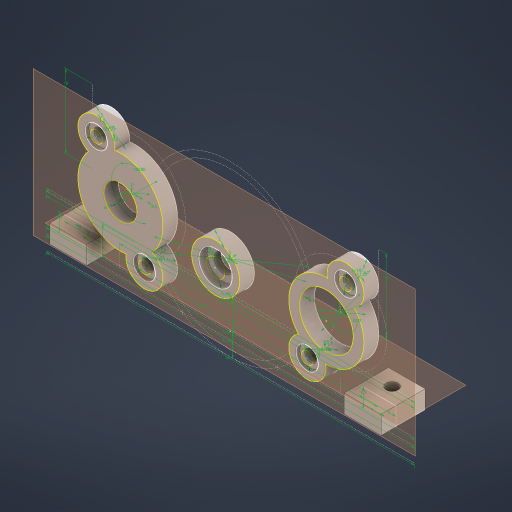
# Autodesk Inventor part: Motormount
Saved by Autodesk Inventor 2023.4 (Build 274418000, 418)
## iProperties
Created: 2024-12-07
Part Number: Motormount
Material: 一般
Document SubType Name: Modeling
Designer: IshiiLabHonda
Density: 1 g/cm^3
Appearance: 既定
Author: IshiiLabHonda
Autodesk Inventor part; units mm, degrees
ref_plane "YZ Plane" through (0, 0, 0) normal (1, 0, 0) x (0, 1, 0)
ref_plane "XZ Plane" through (0, 0, 0) normal (0, 1, 0) x (-1, 0, 0)
ref_plane "XY Plane" through (0, 0, 0) normal (0, 0, 1) x (1, 0, 0)
sketch "blueprint" plane through (0, 0, 0) normal (0, 0, 1) x (1, 0, 0)
  line L0 (0, 0) -> (0, 1) construction
  line L1 (0, 0) -> (1, 0) construction
  circle A0 centre (0, 0) radius 1.25
  circle A1 centre (0, 0) radius 11.5 construction
  line L2 (-25, -11.5) -> (25, -11.5) construction
  line L3 (-25, -9.5) -> (25, -9.5) construction
  line L4 (-25, -8.5) -> (25, -8.5) construction
  line L5 (-25, -4.5) -> (25, -4.5) construction
  circle A2 centre (0, 0) radius 10.65 construction
  circle A3 centre (-12.9388, 1.26) radius 2.25
  circle A4 centre (15.0473, 1.26) radius 4.35 construction
  circle A5 centre (15.0473, 1.26) radius 3.6 construction
  line L6 (-25, -4.1) -> (25, -4.1) construction
  circle A6 centre (-12.9388, 1.26) radius 4.26 construction
  circle A7 centre (-12.9388, 1.26) radius 5.76
  circle A8 centre (-16.1988, 7.3243) radius 0.625 construction
  circle A9 centre (-9.6788, -4.8043) radius 0.625 construction
  circle A10 centre (-12.9388, 1.26) radius 6.885 construction
  circle A11 centre (-16.1988, 7.3243) radius 1.825 construction
  circle A12 centre (-9.6788, -4.8043) radius 1.825 construction
  circle A13 centre (15.0473, 1.26) radius 5.1
  circle A14 centre (15.0473, 1.26) radius 6.225 construction
  circle A15 centre (17.6473, 6.916) radius 0.625 construction
  circle A16 centre (12.4473, -4.396) radius 0.625 construction
  circle A17 centre (17.6473, 6.916) radius 1.825 construction
  circle A18 centre (-16.1988, 7.3243) radius 0.8
  circle A19 centre (-9.6788, -4.8043) radius 0.8
  circle A20 centre (12.4473, -4.396) radius 0.8
  circle A21 centre (17.6473, 6.916) radius 0.8
  circle A22 centre (-16.1988, 7.3243) radius 2.5
  circle A23 centre (-9.6788, -4.8043) radius 2.5
  circle A24 centre (17.6473, 6.916) radius 2.5
  circle A25 centre (12.4473, -4.396) radius 2.5
  circle A26 centre (15.0473, 1.26) radius 3.65
  circle A27 centre (0, 0) radius 3.25
  line L7 (-12.9388, 1.26) -> (-12.9388, 2.26) construction
  line L8 (-12.9388, 1.26) -> (-11.9388, 1.26) construction
  line L9 (15.0473, 1.26) -> (15.0473, 2.26) construction
  line L10 (15.0473, 1.26) -> (16.0473, 1.26) construction
  line L11 (-15, -4.5) -> (-15, -8.5) construction
  line L12 (15, -4.5) -> (15, -8.5) construction
  line L13 (-12.9388, 1.26) -> (15.0473, 1.26) construction
  line L14 (-17.5, -8.5) -> (-17.5, -6)
  line L15 (-22.5, -8.5) -> (-22.5, -6)
  line L16 (-22.5, -6) -> (-17.5, -6)
  line L17 (-20, -6) -> (-20, -8.5)
  line L18 (-21, -6) -> (-21, -8.5)
  line L19 (-19, -6) -> (-19, -8.5)
  line L20 (17.5, -8.5) -> (17.5, -6)
  line L21 (22.5, -8.5) -> (22.5, -6)
  line L22 (22.5, -6) -> (17.5, -6)
  line L23 (20, -6) -> (20, -8.5)
  line L24 (21, -6) -> (21, -8.5)
  line L25 (19, -6) -> (19, -8.5)
  line L26 (-22.5, -8.5) -> (-17.5, -8.5)
  line L27 (17.5, -8.5) -> (22.5, -8.5)
  circle A28 centre (12.4473, -4.396) radius 1.825 construction
  line L28 (-12.9388, 1.26) -> (-16.1988, 7.3243) construction
  line L29 (-12.9388, 1.26) -> (-9.6788, -4.8043) construction
  line L30 (15.0473, 1.26) -> (12.4473, -4.396) construction
  line L31 (-18.6988, 11.26) -> (-18.6988, 1.26) construction
  line L32 (20.1473, 11.26) -> (20.1473, 1.26) construction
  line L33 (17.6473, 6.916) -> (15.0473, 1.26) construction
  point P0 (-8.6127, -2.543)
  point P1 (18.8099, 4.7028)
  point P2 (11.2847, -2.1828)
  point P3 (15.2106, 6.3574)
  point P4 (-12.153, -4.4461)
  point P5 (-13.7246, 6.9661)
  point P6 (14.8841, -3.8374)
  point P7 (-17.2649, 5.063)
  point P8 (0, -8.5)
  point P9 (-6.4807, -9.5)
  point P10 (6.4807, -9.5)
  dimension "d86" = 4
  dimension "d0" = 1
  dimension "d1" = 1
  dimension "d2" = 2.5
  dimension "d3" = 23
  dimension "d4" = 50
  dimension "d5" = 50
  dimension "d6" = 2
  dimension "d7" = 50
  dimension "d9" = 1
  dimension "d10" = 50
  dimension "d12" = 4
  dimension "d13" = 21.3
  dimension "d14" = 4.5
  dimension "d15" = 8.7
  dimension "d17" = 0.1
  dimension "d18" = 0.1
  dimension "d20" = 7.2
  dimension "d21" = 50
  dimension "d22" = 0.4
  dimension "d23" = 8.52
  dimension "d25" = 1.5
  dimension "d26" = 1.25
  dimension "d27" = 1.25
  dimension "d28" = 1.2
  dimension "d29" = 1.2
  dimension "d31" = 1.5
  dimension "d32" = 1.25
  dimension "d33" = 1.25
  dimension "d34" = 1.2
  dimension "d37" = 0.5
  dimension "d39" = 0.5
  dimension "d40" = 1.6
  dimension "d41" = 1.6
  dimension "d42" = 1.6
  dimension "d43" = 1.6
  dimension "d48" = 7.3
  dimension "d49" = 2
  dimension "d50" = 1
  dimension "d51" = 1
  dimension "d52" = 1
  dimension "d53" = 1
  dimension "d56" = 30
  dimension "d90" = 2.5
  dimension "d92" = 5
  dimension "d93" = 2
  dimension "d104" = 1.2
  dimension "d105" = 5
  dimension "d106" = 2
  dimension "d107" = 2.5
  dimension "d128" = 180
  dimension "d129" = 5
  dimension "d130" = 5
  dimension "d131" = 10
  dimension "d132" = 5
  dimension "d133" = 5
  dimension "d134" = 10
  dimension "d135" = 180
  dimension "d155" = 40
  constraints: 66 end point, 27 centre point, 25 coincident, 11 point on line, 11 vertical, 6 parallel, 6 point on circle, 5 symmetric about line, 4 perpendicular, 3 horizontal, 3 midpoint, 3 tangent, 1 collinear, 23 other
  measures "d0" distance of L0.start L0.end
  measures "d1" distance of L0.start L1.end
  measures "d2" diameter of A0
  measures "d3" diameter of A1
  measures "d4" distance of L2.start L2.end
  measures "d5" distance of L3.start L3.end
  measures "d6" distance between parallel lines of L2 L3
  measures "d7" distance of point (-25, -8.5) point (25, -8.5)
  measures "d10" distance of L5.start L5.end
  measures "d13" diameter of A2
  measures "d14" diameter of A3
  measures "d15" diameter of A4
  measures "d20" diameter of A5
  measures "d21" distance of L6.start L6.end
  measures "d22" distance between parallel lines of L5 L6
  measures "d23" diameter of A6
  measures "d26" diameter of A9
  measures "d27" diameter of A8
  measures "d28" radial gap between concentric circles of A11 A8
  measures "d29" radial gap between concentric circles of A12 A9
  measures "d32" diameter of A15
  measures "d33" diameter of A16
  measures "d34" radial gap between concentric circles of A15 A17
  measures "d40" diameter of A18
  measures "d41" diameter of A19
  measures "d42" diameter of A20
  measures "d43" diameter of A21
  measures "d48" diameter of A26
  measures "d49" radial gap between concentric circles of A27 A0
  measures "d50" distance of L7.start L8.end
  measures "d51" distance of L7.start L7.end
  measures "d52" distance of L9.start L9.end
  measures "d53" distance of L9.start L10.end
  measures "d56" distance between parallel lines of L12 L11
  measures "d90" distance of L15.start L15.end
  measures "d92" distance between parallel lines of L14 L15
  measures "d93" distance between parallel lines of L19 L18
  measures "d104" radial gap between concentric circles of A28 A16
  measures "d105" distance between parallel lines of L21 L20
  measures "d106" distance between parallel lines of L24 L25
  measures "d107" distance of L20.start L20.end
  measures "d128" angle of L29 L28
  measures "d129" diameter of A22
  measures "d130" diameter of A23
  measures "d131" distance of L31.start L31.end
  measures "d132" diameter of A24
  measures "d133" diameter of A25
  measures "d134" distance of L32.start L32.end
  measures "d135" angle of L33 L30
  measures "d155" distance between parallel lines of L23 L17
extrude "押し出し18" add sketch "blueprint" along normal blind 2
extrude "押し出し19" add sketch "blueprint" against normal blind 4 contours L26 L19 L16 L14 | L26 L17 L16 L19 | L26 L18 L16 L17 | L26 L15 L16 L18 | L20 L22 L25 L27 | L25 L22 L23 L27 | L23 L22 L24 L27 | L24 L22 L21 L27
ref_plane "作業平面1" through (-22.5, -6, 2) normal (0, 1, 0) x (1, 0, 0)
sketch "スケッチ2" plane through (-22.5, -6, 2) normal (0, 1, 0) x (1, 0, 0)
  line L0 (40, 6) -> (40, 0) projected
  line L1 (45, 0) -> (40, 0) projected
  line L2 (45, 6) -> (45, 0) projected
  line L3 (40, 6) -> (45, 6) projected
  line L4 (0, 6) -> (0, 0) projected
  line L5 (5, 0) -> (0, 0) projected
  line L6 (5, 0) -> (5, 6) projected
  line L7 (0, 6) -> (5, 6) projected
  line L8 (0, 2) -> (5, 2) projected
  line L9 (45, 2) -> (40, 2) projected
  line L10 (0, 6) -> (0, 0) projected
  line L11 (5, 2) -> (0, 6) construction
  line L12 (5, 6) -> (5, 0) projected
  line L13 (5, 6) -> (0, 2) construction
  line L14 (45, 0) -> (45, 6) projected
  line L15 (40, 2) -> (45, 6) construction
  line L16 (40, 6) -> (40, 0) projected
  line L17 (45, 2) -> (40, 6) construction
  circle A0 centre (2.5, 4) radius 0.8
  circle A1 centre (42.5, 4) radius 0.8
  point P0 (22.5, 2)
  dimension "d141" = 1.6
  dimension "d142" = 1.6
  constraints: 8 end point, 2 centre point, 2 midpoint
  measures "d141" diameter of A0
  measures "d142" diameter of A1
extrude "押し出し20" cut sketch "スケッチ2" against normal blind 4 contours A0 | A1
ref_plane "作業平面2" through (0, 0, 2) normal (0, 0, 1) x (1, 0, 0)
sketch "スケッチ3" plane through (0, 0, 2) normal (0, 0, 1) x (1, 0, 0)
  arc A0 (-17.2649, 5.063) -> (-12.153, -4.4461) centre (-12.9388, 1.26) ccw projected
  arc A1 (-12.153, -4.4461) -> (-8.6127, -2.543) centre (-9.6788, -4.8043) ccw projected
  arc A2 (-8.6127, -2.543) -> (-13.7246, 6.9661) centre (-12.9388, 1.26) ccw projected
  arc A3 (-13.7246, 6.9661) -> (-17.2649, 5.063) centre (-16.1988, 7.3243) ccw projected
  circle A4 centre (-9.6788, -4.8043) radius 0.8 projected
  circle A5 centre (-12.9388, 1.26) radius 2.25 projected
  circle A6 centre (-16.1988, 7.3243) radius 0.8 projected
  arc A7 (14.8841, -3.8374) -> (18.8099, 4.7028) centre (15.0473, 1.26) ccw projected
  arc A8 (18.8099, 4.7028) -> (15.2106, 6.3574) centre (17.6473, 6.916) ccw projected
  arc A9 (15.2106, 6.3574) -> (11.2847, -2.1828) centre (15.0473, 1.26) ccw projected
  arc A10 (11.2847, -2.1828) -> (14.8841, -3.8374) centre (12.4473, -4.396) ccw projected
  circle A11 centre (17.6473, 6.916) radius 0.8 projected
  circle A12 centre (15.0473, 1.26) radius 3.65 projected
  circle A13 centre (12.4473, -4.396) radius 0.8 projected
  circle A14 centre (0, 0) radius 3.25 projected
  circle A15 centre (0, 0) radius 1.25 projected
  circle A16 centre (-16.1988, 7.3243) radius 1.5
  circle A17 centre (-9.6788, -4.8043) radius 0.8 projected
  circle A18 centre (-9.6788, -4.8043) radius 1.5
  circle A19 centre (17.6473, 6.916) radius 0.8 projected
  circle A20 centre (17.6473, 6.916) radius 1.5
  circle A21 centre (12.4473, -4.396) radius 0.8 projected
  circle A22 centre (12.4473, -4.396) radius 1.5
  circle A23 centre (0, 0) radius 2.25
  dimension "d146" = 3
  dimension "d147" = 3
  dimension "d148" = 3
  dimension "d149" = 3
  dimension "d150" = 4.5
  constraints: 5 centre point, 5 coincident
  measures "d146" diameter of A16
  measures "d147" diameter of A18
  measures "d148" diameter of A20
  measures "d149" diameter of A22
  measures "d150" diameter of A23
extrude "押し出し21" cut sketch "スケッチ3" against normal blind 1.1 contours A23
extrude "押し出し22" cut sketch "スケッチ3" against normal blind 0.5 contours A16 | A18 | A20 | A22
equation "\"d5\" = d4"
equation "\"d7\" = d4"
equation "\"d10\" = d4"
